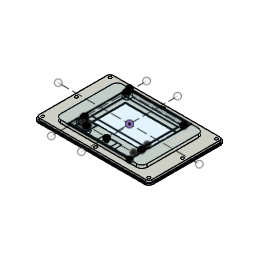
Display Mount - TFT35E3V30 (Autodesk Fusion 360 design; units mm, degrees)
Autodesk Fusion 360 part; units mm, degrees
note: some values were not read from the file. Set by a fixed rule: which sketch regions a step uses.
sketch "Sketch1" plane through (0, 0, 0) normal (0, 0, 1) x (1, 0, 0)
  circle A0 centre (-81.65, 51.9125) radius 2.3
  circle A1 centre (81.65, 51.9125) radius 2.3
  circle A2 centre (-81.65, -51.9125) radius 2.3
  circle A3 centre (81.65, -51.9125) radius 2.3
  line L0 (-81.65, 51.9125) -> (81.65, 51.9125) construction
  line L1 (81.65, 51.9125) -> (81.65, -51.9125) construction
  line L2 (81.65, -51.9125) -> (-81.65, -51.9125) construction
  line L3 (-81.65, -51.9125) -> (-81.65, 51.9125) construction
  circle A4 centre (-81.65, 0) radius 2.3
  circle A5 centre (0, 51.9125) radius 2.3
  circle A6 centre (81.65, 0) radius 2.3
  circle A7 centre (0, -51.9125) radius 2.3
  line L4 (0, 87.0412) -> (0, 82.962)
  line L5 (0, 82.962) -> (0, -82.962) construction
  line L6 (-123.3001, 0) -> (123.3001, 0) construction
  circle A8 centre (81.65, -51.9125) radius 4.9
  circle A9 centre (-81.65, -51.9125) radius 4.9
  circle A10 centre (-81.65, 51.9125) radius 4.9
  circle A11 centre (81.65, 51.9125) radius 4.9
  line L7 (-81.65, 56.8125) -> (81.65, 56.8125)
  line L8 (86.55, 51.9125) -> (86.55, -51.9125)
  line L9 (-81.65, -56.8125) -> (-65.5347, -56.8125)
  line L10 (-65.5347, -56.8125) -> (81.65, -56.8125)
  line L11 (-86.55, 51.9125) -> (-86.55, -51.9125)
  point P0 (0, 51.9125)
  point P1 (81.65, 0)
  point P2 (0, -51.9125)
  point P3 (-81.65, 0)
  dimension "d23" = 4.6
  dimension "d24" = 4.6
  dimension "d25" = 4.6
  dimension "d26" = 4.6
  dimension "d92" = 4.6
  dimension "d93" = 4.6
  dimension "d94" = 4.6
  dimension "d95" = 4.6
  dimension "d178" = 163.3
  dimension "d179" = 103.825
  dimension "d180" = 9.8
  dimension "d181" = 9.8
  dimension "d182" = 9.8
  dimension "d183" = 9.8
  constraint coincident A0.centre L0.start
  constraint coincident A3.centre L1.end
  constraint coincident A2.centre L2.end
  constraint midpoint L0 P0
  constraint midpoint L1 P1
  constraint midpoint L2 P2
  constraint midpoint L3 P3
  constraint coincident P3 A4.centre
  constraint coincident P0 A5.centre
  constraint coincident P1 A6.centre
  constraint coincident P2 A7.centre
  constraint midpoint origin L6
  constraint midpoint origin L5
  constraint symmetric A0.centre A1.centre L5
  constraint vertical A0.centre P3
  constraint symmetric A0.centre A2.centre L6
  constraint coincident P1 L6
  constraint parallel L0 L2
  constraint parallel L1 L3
  constraint coincident P0 L5
  constraint concentric A3 A8
  constraint concentric A2 A9
  constraint concentric A0 A10
  constraint concentric A1 A11
  constraint coincident A10 L7.start
  constraint coincident A11 L7.end
  constraint parallel L0 L7
  constraint tangent A11 L7
  constraint coincident A11 L8.start
  constraint coincident A8 L8.end
  constraint vertical L8
  constraint tangent A8 L8
  constraint coincident A9 L9.start
  constraint tangent A9 L9
  constraint perpendicular L5 L9
  constraint coincident A8 L10.end
  constraint tangent A8 L10
  constraint perpendicular L5 L10
  constraint coincident A10 L11.start
  constraint coincident A9 L11.end
  constraint tangent A9 L11
  constraint tangent A10 L11
  measures "d23" diameter of A0
  measures "d24" diameter of A1
  measures "d25" diameter of A2
  measures "d26" diameter of A3
  measures "d92" diameter of A4
  measures "d93" diameter of A7
  measures "d94" diameter of A6
  measures "d95" diameter of A5
  measures "d178" distance of A0.centre A1.centre
  measures "d179" distance of A0.centre A2.centre
  measures "d180" diameter of A8
  measures "d181" diameter of A9
  measures "d182" diameter of A10
  measures "d183" diameter of A11
extrude "Extrude1" add sketch "Sketch1" along normal blind 3
sketch "Sketch6" plane through (0, 0, 3) normal (0, 0, 1) x (-1, 0, 0)
  circle A0 centre (-81.65, 51.9125) radius 2.3
  circle A1 centre (-81.65, -51.9125) radius 2.3
  circle A2 centre (81.65, -51.9125) radius 2.3
  circle A3 centre (81.65, 51.9125) radius 2.3
  line L0 (0, -100) -> (0, 100) construction
  line L1 (148.8555, 0) -> (144.6445, 0)
  line L2 (144.6445, 0) -> (-144.6445, 0) construction
  line L3 (66.4, -47.3125) -> (-66.4, -47.3125)
  line L4 (-66.4, -47.3125) -> (-66.4, 47.3125)
  line L5 (-66.4, 47.3125) -> (66.4, 47.3125)
  line L6 (66.4, 47.3125) -> (66.4, -47.3125)
  circle A4 centre (0, 51.9125) radius 2.3
  circle A5 centre (81.65, 0) radius 2.3
  circle A6 centre (0, -51.9125) radius 2.3
  circle A7 centre (-81.65, 0) radius 2.3
  arc A8 (-81.65, 56.8125) -> (-86.55, 51.9125) centre (-81.65, 51.9125) ccw
  arc A9 (-86.55, -51.9125) -> (-81.65, -56.8125) centre (-81.65, -51.9125) ccw
  arc A10 (81.65, -56.8125) -> (86.55, -51.9125) centre (81.65, -51.9125) ccw
  arc A11 (86.55, 51.9125) -> (81.65, 56.8125) centre (81.65, 51.9125) ccw
  line L7 (-81.65, -56.8125) -> (81.65, -56.8125)
  line L8 (86.55, -51.9125) -> (86.55, 51.9125)
  line L9 (81.65, 56.8125) -> (-81.65, 56.8125)
  line L10 (-86.55, 51.9125) -> (-86.55, -51.9125)
  dimension "d62" = 66.4
  dimension "d63" = 132.8
  dimension "d64" = 47.3125
  dimension "d65" = 94.625
  constraint vertical L0
  constraint horizontal L1
  constraint midpoint origin L2
  constraint midpoint origin L0
  constraint horizontal L3
  constraint vertical L4
  constraint horizontal L5
  constraint vertical L6
  constraint symmetric L0 L4 L6
  constraint symmetric L2 L3 L5
  measures "d62" distance of L0 L6
  measures "d63" distance of L4 L6
  measures "d64" distance of L2 L5
  measures "d65" distance of L3 L5
extrude "Extrude7" add sketch "Sketch6" along normal blind 4.75 contours L3 L4 L5 L6
fillet "Fillet2" radius 8 4 edges at (-66.4, -47.3125, 5.375) (66.4, -47.3125, 5.375) (66.4, 47.3125, 5.375) (-66.4, 47.3125, 5.375)
sketch "Sketch7" plane through (0, 0, 7.75) normal (0, 0, 1) x (-1, 0, 0)
  arc A0 (58.4, -47.3125) -> (66.4, -39.3125) centre (58.4, -39.3125) ccw
  line L0 (66.4, -39.3125) -> (66.4, 39.3125)
  arc A1 (66.4, 39.3125) -> (58.4, 47.3125) centre (58.4, 39.3125) ccw
  line L1 (58.4, 47.3125) -> (-58.4, 47.3125)
  arc A2 (-58.4, 47.3125) -> (-66.4, 39.3125) centre (-58.4, 39.3125) ccw
  line L2 (-66.4, 39.3125) -> (-66.4, -39.3125)
  arc A3 (-66.4, -39.3125) -> (-58.4, -47.3125) centre (-58.4, -39.3125) ccw
  line L3 (-58.4, -47.3125) -> (58.4, -47.3125)
  line L4 (0, -73.9327) -> (0, 73.9327) construction
  line L5 (109.5416, 0) -> (107.2442, 0)
  line L6 (107.2442, 0) -> (-107.2442, 0) construction
  line L7 (39.5, -33.25) -> (-41.5, -33.25)
  line L8 (-41.5, -33.25) -> (-41.5, 18.25)
  line L9 (-41.5, 18.25) -> (39.5, 18.25)
  line L10 (39.5, 18.25) -> (39.5, -33.25)
  line L11 (39.5, 35.05) -> (-41.5, 35.05) construction
  line L12 (46.5, -44.5) -> (-46.5, -44.5) construction
  line L13 (-46.5, -44.5) -> (-46.5, 44.5) construction
  line L14 (-46.5, 44.5) -> (46.5, 44.5) construction
  line L15 (46.5, 44.5) -> (46.5, -44.5) construction
  line L16 (39, 18.25) -> (39, 33.25) construction
  circle A4 centre (44, -39.5) radius 2.5 construction
  circle A5 centre (-44, -39.5) radius 2.5 construction
  circle A6 centre (44, -39.5) radius 1.4
  circle A7 centre (-44, -39.5) radius 1.4
  circle A8 centre (-44, -39.5) radius 3.5
  circle A9 centre (44, -39.5) radius 3.5
  line L17 (47.5, -47.3125) -> (-47.5, -47.3125)
  line L18 (-47.5, -47.3125) -> (-47.5, 47.3125)
  line L19 (-47.5, 47.3125) -> (47.5, 47.3125)
  line L20 (47.5, 47.3125) -> (47.5, -47.3125)
  line L21 (39, 27.05) -> (23, 27.05)
  line L22 (23, 27.05) -> (23, 43.05)
  line L23 (23, 43.05) -> (39, 43.05)
  line L24 (39, 43.05) -> (39, 27.05)
  line L25 (31, 27.05) -> (31, 43.05) construction
  line L26 (39, 35.05) -> (23, 35.05) construction
  line L27 (-41.5, 14.25) -> (-41.5, -33.25)
  line L28 (47.5, 45.5) -> (-47.5, 45.5)
  line L29 (47.5, -45.5) -> (-47.5, -45.5)
  circle A10 centre (44, 25.5) radius 2.5
  circle A11 centre (44, 25.5) radius 1.4
  circle A12 centre (-44, 25.5) radius 2.5
  circle A13 centre (-44, 25.5) radius 1.4
  circle A14 centre (44, 25.5) radius 3.5
  line L30 (47.5, 17.0503) -> (41.5251, 23.0251)
  line L31 (47.5, 33.9497) -> (41.5251, 27.9749)
  circle A15 centre (-44, 25.5) radius 3.5
  line L32 (-41.5251, 23.0251) -> (-47.5, 17.0503)
  line L33 (-41.5251, 27.9749) -> (-47.5, 33.9497)
  circle A16 centre (31, 35.05) radius 5
  line L34 (40.5, -45.5) -> (40.5, -39.5)
  line L35 (44, -36) -> (47.5, -36)
  line L36 (-44, -36) -> (-47.5, -36)
  line L37 (-40.5, -39.5) -> (-40.5, -45.5)
  line L38 (44, -39.5) -> (-44, -39.5) construction
  circle A17 centre (-1.5, 36.65) radius 2.2
  line L39 (-1.5, 44.5) -> (-1.5, 0) construction
  line L40 (44, 25.5) -> (-44, 25.5) construction
  line L41 (44, -70.3078) -> (44, 76.2367) construction
  point P0 (31, 35.05)
  point P1 (-1.5, 36.65)
  dimension "d96" = 16.8
  dimension "d99" = 44.5
  dimension "d100" = 11.25
  dimension "d101" = 26.25
  dimension "d103" = 5
  dimension "d104" = 5
  dimension "d107" = 2.8
  dimension "d108" = 2.8
  dimension "d113" = 7
  dimension "d114" = 7
  dimension "d116" = 7
  dimension "d121" = 16
  dimension "d123" = 16
  dimension "d134" = 1
  dimension "d135" = 1
  dimension "d136" = 5
  dimension "d137" = 2.8
  dimension "d138" = 5
  dimension "d139" = 2.8
  dimension "d140" = 65
  dimension "d141" = 7
  dimension "d142" = 45
  dimension "d143" = 45
  dimension "d147" = 4
  dimension "d148" = 7
  dimension "d149" = 45
  dimension "d150" = 45
  dimension "d151" = 1
  dimension "d152" = 10
  dimension "d166" = 3.5
  dimension "d167" = 3.5
  dimension "d169" = 5
  dimension "d170" = 69
  dimension "d177" = 8.5
  dimension "d10" = 4.4
  dimension "d13" = 47.5
  dimension "d15" = 32.5
  dimension "d16" = 6
  dimension "d32" = 1.6
  dimension "d53" = 11.15
  dimension "d54" = 45.5
  dimension "d55" = 13
  dimension "d56" = 9.55
  dimension "d58" = 85.5
  dimension "d59" = 4.5
  dimension "d60" = 7.25
  dimension "d61" = 58.75
  constraint perpendicular L1 L4
  constraint perpendicular L0 L5
  constraint perpendicular L2 L6
  constraint midpoint origin L6
  constraint midpoint origin L4
  constraint horizontal L7
  constraint vertical L8
  constraint horizontal L9
  constraint vertical L10
  constraint perpendicular L8 L11
  constraint vertical L8.end L11.end
  constraint vertical L9.end L11.start
  constraint horizontal L12
  constraint vertical L13
  constraint horizontal L14
  constraint vertical L15
  constraint symmetric L6 L12 L14
  constraint coincident L9 L16.start
  constraint perpendicular L9 L16
  constraint horizontal A4.centre A5.centre
  constraint tangent L15 A4
  constraint concentric A4 A6
  constraint concentric A5 A7
  constraint concentric A5 A8
  constraint concentric A4 A9
  constraint horizontal L17
  constraint vertical L18
  constraint horizontal L19
  constraint vertical L20
  constraint coincident L1 L18.end
  constraint coincident L3 L17.start
  constraint tangent A8 L18
  constraint tangent A9 L20
  constraint horizontal L21
  constraint vertical L22
  constraint horizontal L23
  constraint vertical L24
  constraint midpoint L21 L25.start
  constraint midpoint L23 L25.end
  constraint midpoint L24 L26.start
  constraint midpoint L22 L26.end
  constraint coincident L25 P0
  constraint coincident L26 P0
  constraint coincident L11 P0
  constraint collinear L16 L24
  constraint vertical L27
  constraint coincident L20 L28.start
  constraint coincident L18 L28.end
  constraint perpendicular L18 L28
  constraint coincident L20 L29.start
  constraint coincident L18 L29.end
  constraint perpendicular L18 L29
  constraint concentric A10 A11
  constraint tangent L15 A10
  constraint concentric A12 A13
  constraint tangent L13 A12
  constraint horizontal A10.centre A12.centre
  constraint concentric A11 A14
  constraint coincident L20 L30.start
  constraint coincident A14 L30.end
  constraint tangent A14 L30
  constraint coincident L20 L31.start
  constraint coincident A14 L31.end
  constraint tangent A14 L31
  constraint concentric A13 A15
  constraint coincident L18 L32.end
  constraint coincident A15 L33.start
  constraint coincident L18 L33.end
  constraint tangent A15 L32
  constraint tangent A15 L33
  constraint coincident A15 L32.start
  constraint coincident P0 A16.centre
  constraint coincident A9 L34.end
  constraint tangent A9 L34
  constraint perpendicular L12 L34
  constraint coincident A9 L35.start
  constraint tangent A9 L35
  constraint perpendicular L15 L35
  constraint coincident A8 L36.start
  constraint tangent A8 L36
  constraint perpendicular L13 L36
  constraint coincident A8 L37.start
  constraint tangent A8 L37
  constraint perpendicular L12 L37
  constraint coincident L20 L35.end
  constraint coincident L29 L34.start
  constraint coincident L18 L36.end
  constraint coincident L29 L37.end
  constraint coincident A4.centre A6.centre
  constraint coincident A5.centre A7.centre
  constraint coincident L14 L39.start
  constraint coincident L6 L39.end
  constraint perpendicular L6 L39
  constraint coincident P1 L39
  constraint coincident P1 A17.centre
  constraint coincident A10.centre A11.centre
  constraint coincident A12.centre A13.centre
  constraint perpendicular L26 L41
  constraint coincident A10.centre L41
  measures "d96" distance of L9 L11
  measures "d99" distance of L6 L13.end
  measures "d100" distance of L7 L12
  measures "d101" distance of L9 L14
  measures "d103" diameter of A4
  measures "d104" diameter of A5
  measures "d107" diameter of A6
  measures "d108" diameter of A7
  measures "d113" diameter of A8
  measures "d114" diameter of A9
  measures "d116" distance of L10 L15
  measures "d121" distance of L22.end L23.end
  measures "d123" distance of L21 L23
  measures "d134" distance of L14 L28
  measures "d135" distance of L12 L29
  measures "d136" diameter of A10
  measures "d137" diameter of A11
  measures "d138" diameter of A12
  measures "d139" diameter of A13
  measures "d140" distance of A4.centre A10.centre
  measures "d141" diameter of A14
  measures "d142" angle of L20 L30
  measures "d143" angle of L20 L31
  measures "d147" distance of L8.end L27.start
  measures "d148" diameter of A15
  measures "d149" angle of L18 L32
  measures "d150" angle of L18 L33
  measures "d151" distance of L13 L18
  measures "d152" diameter of A16
  measures "d166" distance of A5.centre L18
  measures "d167" distance of A4.centre L20
  measures "d169" distance of L12 L38
  measures "d177" distance of L10 P0
  measures "d10" diameter of A17
  measures "d13" distance of L4 L20
  measures "d15" distance of L25 L39
  measures "d16" distance of L18 L27
  measures "d32" distance of L11 P1
  measures "d53" distance of P1 L40
  measures "d54" distance of P1 L41
  measures "d55" distance of P0 L41
  measures "d56" distance of P0 L40
  measures "d58" distance of L27 L41
  measures "d59" distance of L10 L41
  measures "d60" distance of L9 L40
  measures "d61" distance of L7 L40
extrude "Extrude13" cut sketch "Sketch7" against normal through all contours A16
extrude "Extrude10" cut sketch "Sketch7" against normal blind 8 contours A6 | A7
extrude "Extrude8" cut sketch "Sketch7" against normal blind 7.5 contours A8 A9 L18 L20 L28 L29 A14 L30 L31 A15 L32 L33 L34 L35 L36 L37 | L21 L22 L23 L24 | A11 | A13 | A17
sketch "Sketch8" plane through (0, 0, 0) normal (0, 0, -1) x (1, 0, 0)
  circle A0 centre (81.65, 51.9125) radius 2.3
  circle A1 centre (0, 51.9125) radius 2.3
  circle A2 centre (-81.65, 0) radius 2.3
  circle A3 centre (-81.65, 51.9125) radius 2.3
  circle A4 centre (81.65, -51.9125) radius 2.3
  circle A5 centre (0, -51.9125) radius 2.3
  circle A6 centre (-81.65, -51.9125) radius 2.3
  circle A7 centre (81.65, 0) radius 2.3
  line L0 (81.65, 58.8125) -> (-81.65, 58.8125)
  line L1 (-88.55, 51.9125) -> (-88.55, -51.9125)
  line L2 (-81.65, -58.8125) -> (81.65, -58.8125)
  line L3 (88.55, -51.9125) -> (88.55, 51.9125)
  arc A8 (86.55, 51.9125) -> (81.65, 56.8125) centre (81.65, 51.9125) ccw
  arc A9 (-81.65, 56.8125) -> (-86.55, 51.9125) centre (-81.65, 51.9125) ccw
  arc A10 (-86.55, -51.9125) -> (-81.65, -56.8125) centre (-81.65, -51.9125) ccw
  arc A11 (81.65, -56.8125) -> (86.55, -51.9125) centre (81.65, -51.9125) ccw
  line L4 (86.55, -51.9125) -> (86.55, 51.9125)
  line L5 (81.65, 56.8125) -> (-81.65, 56.8125)
  line L6 (-86.55, 51.9125) -> (-86.55, -51.9125)
  line L7 (-81.65, -56.8125) -> (81.65, -56.8125)
  circle A12 centre (81.65, 51.9125) radius 6.9
  circle A13 centre (-81.65, 51.9125) radius 6.9
  circle A14 centre (-81.65, -51.9125) radius 6.9
  circle A15 centre (81.65, -51.9125) radius 6.9
  circle A16 centre (-44, -39.5) radius 1.4
  circle A17 centre (44, -39.5) radius 1.4
  circle A18 centre (-31, 35.05) radius 5
  dimension "d184" = 2
  dimension "d185" = 2
  dimension "d186" = 2
  dimension "d187" = 2
  constraint concentric A0 A12
  constraint tangent L3 A12
  constraint tangent L0 A13
  constraint tangent L1 A13
  constraint coincident A3.centre A9.centre
  constraint tangent L1 A14
  constraint tangent L2 A14
  constraint coincident A6.centre A10.centre
  constraint tangent L2 A15
  constraint tangent L3 A15
  constraint coincident A4.centre A11.centre
  constraint coincident L0.end A13
  constraint coincident L0.start A12
  constraint coincident L2.end A15
  constraint coincident L2.start A14
  constraint coincident L1.start A13
  constraint coincident L1.end A14
  constraint coincident L3.start A15
  constraint coincident L3.end A12
  measures "d184" distance of L1 L6
  measures "d185" distance of L0 L5
  measures "d186" distance of L3 L4
  measures "d187" distance of L2 L7
extrude "Extrude15" add sketch "Sketch8" along normal blind 3 contours L0 L5 A12 A13 | A8 L4 L5 A12 | A9 L5 L6 A13 | L3 L4 A12 A15 | L4 L5 L6 L7 A12 A13 A14 A15 | A8 L4 L5 A12 | L1 L6 A13 A14 | A9 L5 L6 A13 | A11 L4 L7 A15 | A10 L6 L7 A14 | L2 L7 A14 A15 | A11 L4 L7 A15 | A10 L6 L7 A14 | A16 | A17 | A18
extrude "Extrude17" cut sketch "Sketch7" against normal through all contours A16
extrude "Extrude11" cut sketch "Sketch7" against normal blind 15 contours L7 L8 L9 L10 L27
extrude "Extrude12" cut sketch "Sketch7" against normal blind 6.5 contours L7 L8 L9 L10 L27
extrude "Extrude18" cut sketch "Sketch7" against normal blind 20 contours A17
fillet "Fillet5" radius 1 8 edges at (88.55, 0, -3) (86.529, -56.7915, -3) (0, -58.8125, -3) (-86.529, -56.7915, -3) (-88.55, 0, -3) (-86.529, 56.7915, -3) (0, 58.8125, -3) (86.529, 56.7915, -3)
chamfer "Chamfer9" distance 1.8 angle 45 4 edges at (41.5, 7.5, -3) (1, 33.25, -3) (-39.5, 7.5, -3) (1, -18.25, -3)
sketch "Sketch12" plane through (0, 0, -3) normal (0, 0, -1) x (1, 0, 0)
  line L0 (87.55, -51.9125) -> (87.55, 51.9125)
  arc A0 (87.55, 51.9125) -> (81.65, 57.8125) centre (81.65, 51.9125) ccw
  line L1 (81.65, 57.8125) -> (-81.65, 57.8125)
  arc A1 (-81.65, 57.8125) -> (-87.55, 51.9125) centre (-81.65, 51.9125) ccw
  line L2 (-87.55, 51.9125) -> (-87.55, -51.9125)
  arc A2 (-87.55, -51.9125) -> (-81.65, -57.8125) centre (-81.65, -51.9125) ccw
  line L3 (-81.65, -57.8125) -> (81.65, -57.8125)
  arc A3 (81.65, -57.8125) -> (87.55, -51.9125) centre (81.65, -51.9125) ccw
  circle A4 centre (1.5, 36.65) radius 2.2
  circle A5 centre (-31, 35.05) radius 5
  circle A6 centre (-81.65, 51.9125) radius 2.3
  circle A7 centre (-81.65, -51.9125) radius 2.3
  circle A8 centre (-81.65, 0) radius 2.3
  circle A9 centre (0, -51.9125) radius 2.3
  circle A10 centre (81.65, 51.9125) radius 2.3
  circle A11 centre (81.65, -51.9125) radius 2.3
  circle A12 centre (81.65, 0) radius 2.3
  circle A13 centre (0, 51.9125) radius 2.3
  line L4 (-41.3, 20.05) -> (43.3, 20.05)
  line L5 (43.3, 20.05) -> (43.3, -35.05)
  line L6 (43.3, -35.05) -> (-41.3, -35.05)
  line L7 (-41.3, -35.05) -> (-41.3, 20.05)
  line L8 (11.5, 29.5) -> (-8.5, 29.5)
  line L9 (-8.5, 29.5) -> (-8.5, 43.8)
  line L10 (-8.5, 43.8) -> (11.5, 43.8)
  line L11 (11.5, 43.8) -> (11.5, 29.5)
  line L12 (1.5, 29.5) -> (1.5, 43.8) construction
  line L13 (11.5, 36.65) -> (-8.5, 36.65) construction
  line L14 (47.5, 45.5) -> (-47.5, 45.5)
  dimension "d37" = 20
  dimension "d38" = 16
  constraint horizontal L8
  constraint vertical L9
  constraint horizontal L10
  constraint vertical L11
  constraint midpoint L8 L12.start
  constraint midpoint L10 L12.end
  constraint midpoint L11 L13.start
  constraint midpoint L9 L13.end
  constraint coincident A4.centre L13
  constraint coincident A4.centre L12
  measures "d37" distance of L9.end L10.end
  measures "d38" distance of L8 L14
sketch "Sketch11" plane through (0, 0, 0.25) normal (0, 0, 1) x (-1, 0, 0)
  circle A0 centre (-1.5, 36.65) radius 2.2
  line L0 (-41.5, -33.25) -> (-41.5, 18.25)
  line L1 (-41.5, 18.25) -> (39.5, 18.25)
  line L2 (39.5, 18.25) -> (39.5, -33.25)
  line L3 (39.5, -33.25) -> (-41.5, -33.25)
  circle A1 centre (31, 35.05) radius 5
  arc A2 (-40.5, -39.5) -> (-44, -36) centre (-44, -39.5) ccw
  line L4 (-40.5, -39.5) -> (-40.5, -45.5)
  line L5 (-40.5, -45.5) -> (40.5, -45.5)
  line L6 (40.5, -45.5) -> (40.5, -39.5)
  arc A3 (44, -36) -> (40.5, -39.5) centre (44, -39.5) ccw
  line L7 (44, -36) -> (47.5, -36)
  line L8 (47.5, -36) -> (47.5, 17.0503)
  line L9 (47.5, 17.0503) -> (41.5251, 23.0251)
  arc A4 (41.5251, 27.9749) -> (41.5251, 23.0251) centre (44, 25.5) ccw
  line L10 (41.5251, 27.9749) -> (47.5, 33.9497)
  line L11 (47.5, 33.9497) -> (47.5, 45.5)
  line L12 (47.5, 45.5) -> (-47.5, 45.5)
  line L13 (-47.5, 45.5) -> (-47.5, 33.9497)
  line L14 (-47.5, 33.9497) -> (-41.5251, 27.9749)
  arc A5 (-41.5251, 23.0251) -> (-41.5251, 27.9749) centre (-44, 25.5) ccw
  line L15 (-41.5251, 23.0251) -> (-47.5, 17.0503)
  line L16 (-47.5, 17.0503) -> (-47.5, -36)
  line L17 (-47.5, -36) -> (-44, -36)
  line L18 (8.5, 29.5) -> (8.5, 43.8)
  line L19 (-11.5, 29.5) -> (8.5, 29.5)
  line L20 (-11.5, 43.8) -> (-11.5, 29.5)
  line L21 (8.5, 43.8) -> (-11.5, 43.8)
  line L22 (8.5, 29.5) -> (-11.5, 29.5)
  line L23 (-11.5, 29.5) -> (-11.5, 43.8)
  line L24 (-11.5, 43.8) -> (8.5, 43.8)
  line L25 (8.5, 43.8) -> (8.5, 29.5)
  constraint horizontal L22
  constraint vertical L23
  constraint horizontal L24
  constraint vertical L25
  constraint coincident L20.start L21.end
  constraint coincident L18.start L19.end
extrude "Extrude22" add sketch "Sketch11" along normal blind 3 contours L18 L19 L20 L21 L22 L23 L24 L25
chamfer "Chamfer11" distance 3 angle 45 3 edges at (11.5, -36.65, 0.25) (1.5, -29.5, 0.25) (-8.5, -36.65, 0.25)
extrude "Extrude23" add 1 faces at (4.8333, -43.8, 1.2498) along direction (0, -1, 0) blind 3.5
sketch "Sketch13" plane through (0, 0, -3) normal (0, 0, -1) x (1, 0, 0)
  line L0 (87.55, -51.9125) -> (87.55, 51.9125)
  arc A0 (87.55, 51.9125) -> (81.65, 57.8125) centre (81.65, 51.9125) ccw
  line L1 (81.65, 57.8125) -> (-81.65, 57.8125)
  arc A1 (-81.65, 57.8125) -> (-87.55, 51.9125) centre (-81.65, 51.9125) ccw
  line L2 (-87.55, 51.9125) -> (-87.55, -51.9125)
  arc A2 (-87.55, -51.9125) -> (-81.65, -57.8125) centre (-81.65, -51.9125) ccw
  line L3 (-81.65, -57.8125) -> (81.65, -57.8125)
  arc A3 (81.65, -57.8125) -> (87.55, -51.9125) centre (81.65, -51.9125) ccw
  circle A4 centre (1.5, 36.65) radius 2.2
  circle A5 centre (-31, 35.05) radius 5
  circle A6 centre (-81.65, 51.9125) radius 2.3
  circle A7 centre (-81.65, -51.9125) radius 2.3
  circle A8 centre (-81.65, 0) radius 2.3
  circle A9 centre (0, -51.9125) radius 2.3
  circle A10 centre (81.65, 51.9125) radius 2.3
  circle A11 centre (81.65, -51.9125) radius 2.3
  circle A12 centre (81.65, 0) radius 2.3
  circle A13 centre (0, 51.9125) radius 2.3
  line L4 (-41.3, 20.05) -> (43.3, 20.05)
  line L5 (43.3, 20.05) -> (43.3, -35.05)
  line L6 (43.3, -35.05) -> (-41.3, -35.05)
  line L7 (-41.3, -35.05) -> (-41.3, 20.05)
extrude "Extrude24" cut sketch "Sketch12" against normal blind 4.4 contours L8 L9 L10 L11
chamfer "Chamfer13" distance 4.4 angle 45 4 edges at (1.5, -29.5, 1.4) (11.5, -36.65, 1.4) (1.5, -43.8, 1.4) (-8.5, -36.65, 1.4)
equation "d24 = d23"
equation "d25 = d23"
equation "d26 = d23"
equation "d92 = d23"
equation "d93 = d23"
equation "d94 = d23"
equation "d95 = d23"
equation "d99 = ( 89 / 2 ) * 1 mm"
equation "d108 = d107"
equation "d113 = d111"
equation "d114 = d111"
equation "d121 = d123"
equation "d137 = d107"
equation "d139 = d107"
equation "d178 = 173.2 mm - 9.9 mm"
equation "d180 = d181"
equation "d182 = d181"
equation "d183 = d181"
equation "d111 = 7 mm"
